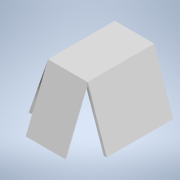
# Autodesk Inventor part: chasis
Saved by Autodesk Inventor 2021 (Build 250183000, 183)
## iProperties
Created: 2021-02-05
Part Number: chasis
Material: Genérico
Document SubType Name: Modeling
Designer: jaime
Density: 1 g/cm^3
Appearance: Valor por defecto
Author: jaime
Autodesk Inventor part; units mm, degrees
ref_plane "YZ Plane" through (0, 0, 0) normal (1, 0, 0) x (0, 1, 0)
ref_plane "XZ Plane" through (0, 0, 0) normal (0, 1, 0) x (-1, 0, 0)
sketch "Boceto1" plane through (0, 0, 0) normal (0, 0, 1) x (1, 0, 0)
  line L0 (0, 0) -> (70.9542, 0)
  line L1 (70.9542, 0) -> (140, -200)
  line L2 (140, -200) -> (0, -200)
  line L3 (0, -200) -> (0, 0) construction
  line L4 (0, 0) -> (-70.9542, 0)
  line L5 (-70.9542, 0) -> (-140, -200)
  line L6 (-140, -200) -> (0, -200)
  dimension "d0" = 280
  dimension "d1" = 200
  constraints: 14 end point, 2 symmetric about line, 1 horizontal, 1 parallel, 1 perpendicular
  measures "d0" distance of L1.end L6.start
  measures "d1" distance between parallel lines of L6 L4
extrude "Extrusión1" add sketch "Boceto1" along normal mid plane 240
sketch "Boceto2" plane through (0, 0, -120) normal (0, 0, -1) x (-1, 0, 0)
  line L0 (-63.8273, -10) -> (63.8273, -10)
  line L1 (140, -200) -> (-140, -200) projected
  line L2 (-63.8273, -10) -> (-129.4209, -200)
  line L3 (63.8273, -10) -> (129.4209, -200)
  line L4 (70.9542, 0) -> (-70.9542, 0) projected
  line L5 (140, -200) -> (70.9542, 0) projected
  line L6 (-70.9542, 0) -> (-140, -200) projected
  point P0 (0, 0)
  dimension "d4" = 10
  dimension "d7" = 10
  dimension "d8" = 10
  constraints: 6 end point, 3 parallel, 2 point on line
  measures "d4" distance between parallel lines of L0 L4
  measures "d7" distance between parallel lines of L5 L3
  measures "d8" distance between parallel lines of L2 L6
extrude "Extrusión2" cut sketch "Boceto2" against normal blind 240 contours L0 L3 L1 L2
ref_plane "Plano de trabajo2" through (0, 205.5279, 120) normal (1, 0, 0) x (0, 0, -1)
sketch "Boceto4" plane through (0, 205.5279, 120) normal (1, 0, 0) x (0, 0, -1)
  line L0 (240, -205.5279) -> (0, -205.5279) projected
  line L1 (0, -205.5279) -> (-80, -405.5279)
  line L2 (-80, -405.5279) -> (-76, -405.5279)
  line L3 (0, -405.5279) -> (0, -205.5279)
  line L4 (0, -215.5279) -> (-76, -405.5279)
  line L5 (0, -215.5279) -> (0, -205.5279)
  line L6 (240, -215.5279) -> (0, -215.5279) projected
  line L7 (0, -215.5279) -> (0, -205.5279)
  line L8 (-80, -405.5279) -> (0, -405.5279) construction
  point P0 (120, -205.5279)
  dimension "d11" = 80
  dimension "d14" = 200
  constraints: 14 end point, 2 collinear, 2 parallel, 2 perpendicular
  measures "d11" distance of L1.end L3.start
  measures "d14" distance between parallel lines of L0 L8
extrude "Extrusión3" add sketch "Boceto4" along normal mid plane 141.908
